# Autodesk Inventor part: spin4v23.brd_Outline1
Saved by Autodesk Inventor 2015 SP1 (Build 190203100, 203)
## iProperties
Created: 2015-06-25
Part Number: spin4v23.brd_Outline1
Material: Generic
Document SubType Name: Modeling
Designer: Patrick
Density: 1 g/cm^3
Appearance: Board Outline
Author: Patrick
Autodesk Inventor part; units mm, degrees
ref_plane "YZ Plane" through (0, 0, 0) normal (1, 0, 0) x (0, 1, 0)
ref_plane "XZ Plane" through (0, 0, 0) normal (0, 1, 0) x (-1, 0, 0)
ref_plane "XY Plane" through (0, 0, 0) normal (0, 0, 1) x (1, 0, 0)
sketch "Sketch1" plane through (0, 0, 0) normal (0, 0, 1) x (1, 0, 0)
  line L0 (-120, -126.7) -> (-120, 126.7)
  line L1 (-120, 126.7) -> (110, 126.7)
  line L2 (110, 126.7) -> (110, -126.7)
  line L3 (110, -126.7) -> (-120, -126.7)
  constraints: 8 end point
extrude "spin4v23.brd_Outline" add sketch "Sketch1" along normal blind 2.508
body "Solid1"
